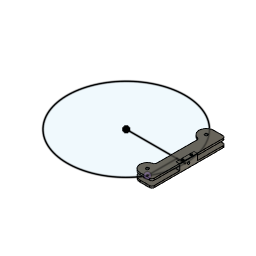
Adaptive_spool_holder_AB _V3 (Autodesk Fusion 360 design; units mm, degrees)
Autodesk Fusion 360 part; units mm, degrees
sketch "Sketch1" plane through (0, 0, 0) normal (0, 0, 1) x (1, 0, 0)
  circle A0 centre (0, 0) radius 4
  dimension "d9" = 8
  constraint coincident A0.centre origin
  measures "d9" diameter of A0
extrude "Extrude1" add sketch "Sketch1" along normal blind 3.4 makes body 1
sketch "Sketch2" plane through (0, 0, 0) normal (0, 0, -1) x (1, 0, 0)
  circle A0 centre (0, 0) radius 4
  circle A1 centre (0, 0) radius 5.5
  dimension "d12" = 11
  constraint coincident A0.centre A1.centre
  measures "d12" diameter of A1
extrude "Extrude2" add sketch "Sketch2" along normal blind 0.5 contours A0 | A1 bodies 1
sketch "Sketch3" plane through (0, 0, -0.5) normal (0, 0, -1) x (1, 0, 0)
  circle A0 centre (0, 0) radius 5.5
  circle A1 centre (0, 0) radius 12.5
  line L0 (0, 0) -> (0, -12.5)
  line L1 (0, 0) -> (0, 12.5)
  line L2 (0, 12.5) -> (20, 12.5)
  line L3 (20, 12.5) -> (20, 0)
  line L4 (0, 0) -> (0, -50)
  line L5 (20, 0) -> (20, -50)
  line L6 (20, -50) -> (0, -50)
  dimension "d17" = 25
  dimension "d18" = 20
  dimension "d19" = 12.5
  dimension "d20" = 50
  dimension "d21" = 50
  constraint concentric A0 A1
  constraint coincident A0.centre A1.centre
  constraint coincident A1 L0.end
  constraint vertical L0
  constraint coincident A1 L1.end
  constraint parallel L0 L1
  constraint tangent A1 L2
  constraint perpendicular L2 L3
  constraint parallel L0 L4
  constraint parallel L3 L5
  measures "d17" diameter of A1
  measures "d18" distance of L1.end L2.end
  measures "d19" distance of L2.end L3.end
  measures "d20" distance of A0.centre L4.end
  measures "d21" distance of L3.end L5.end
extrude "Extrude3" add sketch "Sketch3" along normal blind 3 bodies 1
fillet "Fillet1" radius 4 1 edges at (20, -12.5, -2) on bodies 1
fillet "Fillet2" radius 4 1 edges at (0, 12.5, -2) on bodies 1
mirror "Mirror2" about plane through (20, 50, -0.5) normal (0, 1, 0) of bodies 1 merged
mirror "Mirror4" about plane through (0, 0, 3.4) normal (0, 0, 1) of bodies 1 makes body 2
sketch "Sketch6" plane through (0, 0, -0.5) normal (0, 0, 1) x (-1, 0, 0)
  circle A0 centre (0, -100) radius 5.5
  circle A1 centre (0, 0) radius 5.5
  arc A2 (-16, 12.5) -> (-20, 8.5) centre (-16, 8.5) ccw
  line L0 (-20, 8.5) -> (-20, -108.5)
  arc A3 (-20, -108.5) -> (-16, -112.5) centre (-16, -108.5) ccw
  line L1 (-16, -112.5) -> (0, -112.5)
  arc A4 (0, -112.5) -> (3.0303, -87.8729) centre (0, -100) ccw
  arc A5 (0, -83.9922) -> (3.0303, -87.8729) centre (4, -83.9922) ccw
  line L2 (0, -83.9922) -> (0, -16.0078)
  arc A6 (3.0303, -12.1271) -> (0, -16.0078) centre (4, -16.0078) ccw
  arc A7 (3.0303, -12.1271) -> (0, 12.5) centre (0, 0) ccw
  line L3 (0, 12.5) -> (-16, 12.5)
  line L4 (0, 0) -> (0, -50)
  line L5 (0, -50) -> (-20, -50)
  line L6 (-20, -50) -> (-20, -65)
  line L7 (-20, -65) -> (-14, -65)
  line L8 (-14, -65) -> (-14, -35)
  line L9 (-14, -35) -> (-20, -35)
  line L10 (-20, -35) -> (-20, -65)
  dimension "d48" = 50
  dimension "d49" = 20
  dimension "d50" = 15
  dimension "d51" = 6
  dimension "d52" = 30
  constraint coincident A1.centre A7.centre
  constraint parallel L2 L4
  constraint perpendicular L0 L5
  constraint perpendicular L5 L6
  constraint horizontal L7
  constraint vertical L8
  constraint horizontal L9
  constraint vertical L10
  measures "d48" distance of A1.centre L4.end
  measures "d49" distance of L4.end L5.end
  measures "d50" distance of L5.end L6.end
  measures "d51" distance of L6.end L7.end
  measures "d52" distance of L6.end L9.end
extrude "Extrude5" add sketch "Sketch6" along normal blind 9.8 contours L0 L5 L8 L9 L10 | L0 L5 L6 L7 L8 L10 bodies 1
sketch "Sketch7" plane through (0, 0, 7.3) normal (0, 0, -1) x (1, 0, 0)
  circle A0 centre (0, -100) radius 5.5
  circle A1 centre (0, 0) radius 5.5
  arc A2 (20, 8.5) -> (16, 12.5) centre (16, 8.5) ccw
  line L0 (16, 12.5) -> (0, 12.5)
  arc A3 (0, 12.5) -> (-3.0303, -12.1271) centre (0, 0) ccw
  arc A4 (0, -16.0078) -> (-3.0303, -12.1271) centre (-4, -16.0078) ccw
  line L1 (0, -16.0078) -> (0, -83.9922)
  arc A5 (-3.0303, -87.8729) -> (0, -83.9922) centre (-4, -83.9922) ccw
  arc A6 (-3.0303, -87.8729) -> (0, -112.5) centre (0, -100) ccw
  line L2 (0, -112.5) -> (16, -112.5)
  arc A7 (16, -112.5) -> (20, -108.5) centre (16, -108.5) ccw
  line L3 (20, -108.5) -> (20, 8.5)
  line L4 (0, 0) -> (0, -50)
  line L5 (0, -50) -> (20, -50)
  line L6 (20, -50) -> (20, -65.2)
  line L7 (20, -65.2) -> (13.8, -65.2)
  line L8 (13.8, -65.2) -> (13.8, -34.8)
  line L9 (13.8, -34.8) -> (20, -34.8)
  line L10 (20, -34.8) -> (20, -65.2)
  dimension "d55" = 50
  dimension "d56" = 20
  dimension "d57" = 15.2
  dimension "d58" = 6.2
  dimension "d59" = 30.4
  constraint coincident A1.centre A3.centre
  constraint parallel L1 L4
  constraint perpendicular L4 L5
  constraint perpendicular L5 L6
  constraint horizontal L7
  constraint vertical L8
  constraint horizontal L9
  constraint vertical L10
  measures "d55" distance of A1.centre L4.end
  measures "d56" distance of L4.end L5.end
  measures "d57" distance of L5.end L6.end
  measures "d58" distance of L6.end L7.end
  measures "d59" distance of L6.end L9.end
extrude "Extrude6" cut sketch "Sketch7" against normal blind 2.2 contours L3 L5 L8 L9 L10 | L3 L5 L6 L7 L8 L10 bodies 2
sketch "Sketch8" plane through (0, 0, 10.3) normal (0, 0, 1) x (-1, 0, 0)
  arc A0 (-16, 12.5) -> (-20, 8.5) centre (-16, 8.5) ccw
  line L0 (-20, 8.5) -> (-20, -108.5)
  arc A1 (-20, -108.5) -> (-16, -112.5) centre (-16, -108.5) ccw
  line L1 (-16, -112.5) -> (0, -112.5)
  arc A2 (0, -112.5) -> (3.0303, -87.8729) centre (0, -100) ccw
  arc A3 (0, -83.9922) -> (3.0303, -87.8729) centre (4, -83.9922) ccw
  line L2 (0, -83.9922) -> (0, -16.0078)
  arc A4 (3.0303, -12.1271) -> (0, -16.0078) centre (4, -16.0078) ccw
  arc A5 (3.0303, -12.1271) -> (0, 12.5) centre (0, 0) ccw
  line L3 (0, 12.5) -> (-16, 12.5)
  line L4 (0, 0) -> (-20, 0)
  line L5 (-20, 0) -> (-20, -50)
  line L6 (-20, -50) -> (-17, -50)
  line L7 (-17, -50) -> (-17, -42.5)
  line L8 (-17, -50) -> (-17, -57.5)
  dimension "d63" = 20
  dimension "d64" = 50
  dimension "d65" = 3
  dimension "d66" = 7.5
  dimension "d67" = 7.5
  constraint coincident A5.centre L4.start
  constraint perpendicular L0 L4
  constraint perpendicular L4 L5
  constraint perpendicular L5 L6
  constraint perpendicular L6 L7
  constraint perpendicular L6 L8
  measures "d63" distance of A5.centre L4.end
  measures "d64" distance of L4.end L5.end
  measures "d65" distance of L5.end L6.end
  measures "d66" distance of L6.end L7.end
  measures "d67" distance of L6.end L8.end
hole "Hole1" at (17, 42.5, 10.3) at (17, 57.5, 10.3) direction (0, 0, -1) diameter 3 depth 10 tip angle 118 countersink diameter 4 countersink angle 90 bodies 1 2
sketch "Sketch9" plane through (20, 0, 0) normal (1, 0, 0) x (0, 1, 0)
  line L0 (-8.5, -0.5) -> (-8.5, -3.5)
  line L1 (-8.5, -3.5) -> (108.5, -3.5)
  line L2 (108.5, -3.5) -> (108.5, -0.5)
  line L3 (108.5, -0.5) -> (65, -0.5)
  line L4 (65, -0.5) -> (65, 9.3)
  line L5 (65, 9.3) -> (35, 9.3)
  line L6 (35, 9.3) -> (35, -0.5)
  line L7 (35, -0.5) -> (-8.5, -0.5)
  line L8 (0, 0) -> (50, 0)
  line L9 (50, 0) -> (50, 3.4)
  dimension "d76" = 50
  dimension "d77" = 3.4
  constraint coincident L8.start origin
  constraint parallel L7 L8
  constraint perpendicular L8 L9
  measures "d76" distance of L8.start L8.end
  measures "d77" distance of L8.end L9.end
hole "Hole2" at (20, 50, 3.4) direction (-1, 0, 0) diameter 4 depth 10 tip angle 118 bodies 1
sketch "Sketch10" plane through (14, 0, 0) normal (-1, 0, 0) x (0, -1, 0)
  circle A0 centre (-50, 3.4) radius 2
  line L0 (-65, -0.5) -> (-35, -0.5)
  line L1 (-35, -0.5) -> (-35, 9.3)
  line L2 (-35, 9.3) -> (-65, 9.3)
  line L3 (-65, 9.3) -> (-65, -0.5)
  line L4 (0, 0) -> (-50, 0)
  line L5 (-50, 0) -> (-50, 3.4)
  line L6 (-52.0207, 6.9) -> (-54.0415, 3.4)
  line L7 (-54.0415, 3.4) -> (-52.0207, -0.1)
  line L8 (-52.0207, -0.1) -> (-47.9793, -0.1)
  line L9 (-47.9793, -0.1) -> (-45.9585, 3.4)
  line L10 (-45.9585, 3.4) -> (-47.9793, 6.9)
  line L11 (-47.9793, 6.9) -> (-52.0207, 6.9)
  point P0 (-50, 3.4)
  dimension "d86" = 50
  dimension "d87" = 3.4
  dimension "d88" = 3.5
  constraint coincident L4.start origin
  constraint perpendicular L1 L4
  constraint perpendicular L4 L5
  constraint coincident P0 A0.centre
  measures "d86" distance of L4.start L4.end
  measures "d87" distance of L4.end P0
  measures "d88" distance of P0 L11
extrude "Extrude7" cut sketch "Sketch10" against normal blind 3 contours L6 L7 L8 L9 L10 L11 bodies 1
sketch "Sketch19" plane through (0, 0, 0) normal (0, 0, 1) x (1, 0, 0)
  line L0 (0, 0) -> (0, 50)
  line L1 (0, 50) -> (14, 50)
  line L2 (14, 50) -> (-86, 50)
  circle A0 centre (-86, 50) radius 100
  dimension "d98" = 50
  dimension "d99" = 100
  dimension "d100" = 200
  dimension "d101" = 14
  constraint coincident L0.start origin
  constraint vertical L0
  constraint perpendicular L0 L1
  constraint perpendicular L0 L2
  constraint coincident L2.end A0.centre
  measures "d98" distance of L0.start L0.end
  measures "d99" distance of L1.end L2.end
  measures "d100" diameter of A0
  measures "d101" distance of L0.end L1.end
sketch "Sketch20" plane through (0, 0, 10.3) normal (0, 0, 1) x (-1, 0, 0)
  circle A0 centre (-17, -42.5) radius 2
  circle A1 centre (-17, -57.5) radius 2
  arc A2 (-16, 12.5) -> (-20, 8.5) centre (-16, 8.5) ccw
  line L0 (-20, 8.5) -> (-20, -108.5)
  arc A3 (-20, -108.5) -> (-16, -112.5) centre (-16, -108.5) ccw
  line L1 (-16, -112.5) -> (0, -112.5)
  arc A4 (0, -112.5) -> (3.0303, -87.8729) centre (0, -100) ccw
  arc A5 (0, -83.9922) -> (3.0303, -87.8729) centre (4, -83.9922) ccw
  line L2 (0, -83.9922) -> (0, -16.0078)
  arc A6 (3.0303, -12.1271) -> (0, -16.0078) centre (4, -16.0078) ccw
  arc A7 (3.0303, -12.1271) -> (0, 12.5) centre (0, 0) ccw
  line L3 (0, 12.5) -> (-16, 12.5)
  line L4 (0, 0) -> (0, -100)
  dimension "d102" = 100
  constraint coincident A7.centre L4.start
  constraint parallel L2 L4
  measures "d102" distance of A7.centre A4.centre
hole "Hole3" at (0, 0, 10.3) at (0, 100, 10.3) direction (0, 0, -1) diameter 4 depth 10.8 tip angle 118 countersink diameter 5 countersink angle 90 bodies 1 2
equation "bearring_poke_diameter = 8 mm"
equation "bearring_spacer_diameter = 11 mm"
equation "bearring_poke_height = 3.4 mm"
equation "bearring_spacer_height = 0.5 mm"
equation "bearring_distance_between = 100 mm"
equation "bearring_distance_plane = 20 mm"
equation "plane_thickness = 3 mm"
equation "plane_screw_holes = 3 mm"
equation "d9 = bearring_poke_diameter"
equation "d10 = bearring_poke_height"
equation "d12 = bearring_spacer_diameter"
equation "d13 = bearring_spacer_height"
equation "plate_circle_diameter = 25 mm"
equation "plate_circle_fillet = 4 mm"
equation "d17 = plate_circle_diameter"
equation "d18 = bearring_distance_plane"
equation "d19 = plate_circle_diameter / 2"
equation "d20 = bearring_distance_between / 2"
equation "d21 = bearring_distance_between / 2"
equation "d22 = plane_thickness"
equation "d25 = plate_circle_fillet"
equation "d27 = plate_circle_fillet"
equation "screwplate_length = 40 mm"
equation "screwplate_width = 30 mm"
equation "screwplate_thickness = 6 mm"
equation "screwplate_height = ( bearring_spacer_height + bearring_poke_height ) * 2 + screwplate_height_insert"
equation "screwplate_height_insert = 2 mm"
equation "d48 = bearring_distance_between / 2"
equation "d49 = bearring_distance_plane"
equation "d50 = screwplate_width / 2"
equation "d51 = screwplate_thickness"
equation "d52 = screwplate_width"
equation "d53 = screwplate_height"
equation "d55 = bearring_distance_between / 2"
equation "d56 = bearring_distance_plane"
equation "d57 = screwplate_width / 2 + insert_clearence"
equation "d58 = screwplate_thickness + insert_clearence"
equation "d59 = screwplate_width + ( insert_clearence * 2 )"
equation "d60 = -screwplate_height_insert - insert_clearence"
equation "insert_clearence = 0.2 mm"
equation "d63 = bearring_distance_plane"
equation "d64 = bearring_distance_between / 2"
equation "d65 = screwplate_thickness / 2"
equation "d66 = screwplate_width / 4"
equation "d67 = screwplate_width / 4"
equation "d68 = screw_length"
equation "d69 = screw_size_M"
equation "screw_size_M = 3 mm"
equation "screw_length = 10 mm"
equation "screw_edge_size_M = 4 mm"
equation "d74 = screw_edge_size_M"
equation "d76 = bearring_distance_between / 2"
equation "d77 = bearring_poke_height"
equation "d78 = screw_attach_length"
equation "d79 = screw_attach_size_M"
equation "screw_attach_size_M = 4 mm"
equation "screw_attach_length = 10 mm"
equation "screw_attach_edge_size_M = 5 mm"
equation "d84 = screw_attach_edge_size_M"
equation "d87 = bearring_poke_height"
equation "d88 = screw_attach_nut_size"
equation "screw_attach_nut_size = ( 7 mm / 2 mm ) * 1 mm"
equation "screw_attach_nut_depth = 3 mm"
equation "d91 = -screw_attach_nut_depth"
equation "test_spool_diameter = 200 mm"
equation "d98 = bearring_distance_between / 2"
equation "d99 = test_spool_diameter / 2"
equation "d100 = test_spool_diameter"
equation "d101 = bearring_distance_plane - screwplate_thickness"
equation "d102 = bearring_distance_between"
equation "d103 = plane_thickness + ( bearring_poke_height * 2 ) + ( bearring_spacer_height * 2 )"
equation "d104 = screw_attach_size_M"
equation "d106 = screw_attach_edge_size_M"
named bodies: "Holder_A", "Holder_B"
